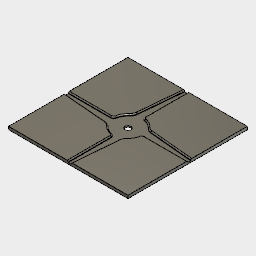
Box Top v3 (Autodesk Fusion 360 design; units mm, degrees)
Autodesk Fusion 360 part; units mm, degrees
sketch "Sketch1" plane through (0, 0, 0) normal (0, 1, 0) x (1, 0, 0)
  line L0 (60, -60) -> (-60, -60)
  line L1 (-60, -60) -> (-60, 60)
  line L2 (-60, 60) -> (60, 60)
  line L3 (60, 60) -> (60, -60)
  line L4 (60, -60) -> (-60, 60) construction
  line L5 (-60, -60) -> (60, 60) construction
  constraint perpendicular L0 L1
  constraint parallel L0 L2
  constraint parallel L1 L3
  constraint horizontal L0
  constraint coincident L4
  constraint coincident L5
extrude "Extrude1" add sketch "Sketch1" along normal blind 3
sketch "Sketch2" plane through (0, 3, 0) normal (0, 1, 0) x (-1, 0, 0)
  line L0 (-60, -60) -> (60, -60)
  line L1 (60, -60) -> (60, 60)
  line L2 (60, 60) -> (-60, 60)
  line L3 (-60, 60) -> (-60, -60)
  circle A0 centre (0, 0) radius 3
  line L4 (0, -60) -> (0, -17.2409)
  line L5 (60, 0) -> (17.4152, 0)
  line L6 (0, 60) -> (0, 16.9303)
  line L7 (-60, 0) -> (-16.7383, 0)
  line L8 (-60, -60) -> (60, -60)
  line L9 (3, -60) -> (7.0006, -16.2997)
  line L10 (60, -60) -> (60, 60)
  line L11 (60, 60) -> (-60, 60)
  line L12 (-60, 60) -> (-60, -60)
  line L13 (-60, -3) -> (-16.05, -7.0235)
  line L14 (60, 3) -> (15.8991, 6.7805)
  line L15 (-2.8992, 60) -> (-6.6949, 15.7222)
  arc A1 (-9.3339, 10.4412) -> (-13.7854, 2.4707) centre (0, 0) ccw
  arc A2 (10.6052, 9.4341) -> (2.4766, 13.9763) centre (0, 0) ccw
  arc A3 (-10.8133, -9.6603) -> (-2.4857, -14.2853) centre (0, 0) ccw
  arc A4 (9.6859, -11.0201) -> (14.4588, -2.4907) centre (0, 0) ccw
  arc A5 (10.6052, 9.4341) -> (15.8991, 6.7805) centre (16.5824, 14.7513) ccw
  arc A6 (9.6859, -11.0201) -> (7.0006, -16.2997) centre (14.9673, -17.029) ccw
  arc A7 (-10.8133, -9.6603) -> (-16.05, -7.0235) centre (-16.7793, -14.9902) ccw
  arc A8 (-9.3339, 10.4412) -> (-6.6949, 15.7222) centre (-14.6657, 16.4055) ccw
  arc A9 (0, -17.2409) -> (-2.4857, -14.2853) centre (-3, -17.2409) ccw
  arc A10 (-16.7383, 0) -> (-13.7854, 2.4707) centre (-16.7383, 3) ccw
  arc A11 (0, 16.9303) -> (2.4766, 13.9763) centre (3, 16.9303) ccw
  arc A12 (17.4152, 0) -> (14.4588, -2.4907) centre (17.4152, -3) ccw
  dimension "d3" = 6
  dimension "d4" = 29
  dimension "d5" = 3
  dimension "d8" = 3
  dimension "d12" = 3
  dimension "d15" = 8
  dimension "d16" = 3
  constraint concentric A0 A3
  constraint midpoint L0
  constraint perpendicular L0 L4
  constraint midpoint L1
  constraint perpendicular L1 L5
  constraint midpoint L2
  constraint perpendicular L2 L6
  constraint midpoint L3
  constraint perpendicular L3 L7
  constraint coincident L0
  constraint coincident L3
  constraint coincident L10
  constraint coincident L11
  constraint perpendicular L14 L15
  constraint concentric A1 A3
  constraint concentric A2 A3
  constraint concentric A3 A4
  constraint tangent L14 A5
  constraint tangent A2 A5
  constraint tangent L9 A6
  constraint tangent A4 A6
  constraint equal A5 A6
  constraint tangent L13 A7
  constraint tangent A3 A7
  constraint equal A5 A7
  constraint tangent L15 A8
  constraint tangent A1 A8
  constraint equal A5 A8
  constraint tangent L4 A9
  constraint tangent A3 A9
  constraint tangent L7 A10
  constraint tangent A1 A10
  constraint equal A9 A10
  constraint tangent L6 A11
  constraint tangent A2 A11
  constraint equal A9 A11
  constraint tangent L5 A12
  constraint tangent A4 A12
  constraint equal A9 A12
  measures "d3" diameter of A0
  measures "d4" diameter of A3
  measures "d15" radius of A5
  measures "d16" radius of A9
extrude "Extrude2" cut sketch "Sketch2" against normal blind 1.5 contours L0 L1 L2 L3 L4 L5 L6 L7 L8 L9 L10 L11 L12 L13 L14 L15 A1 A2 A3 A4 A5 A6 A7 A8 A9 A10 A11 A12
extrude "Extrude3" cut 1 faces at (0.9888, 3, 0.149) along direction (0, -1, 0) blind 10
fillet "Fillet1" radius 1 20 edges at (-38.7076, 3, 0) (-15.4823, 3, -0.7057) (-12.8035, 3, -7.1645) (-7.8366, 3, -13.4022) (-5.0003, 3, -38.1498) (0, 3, 38.4652) (-0.7011, 3, 15.0029) (-6.9239, 3, 12.3907) (-12.9976, 3, 7.5994) (-37.9496, 3, 4.8902) (38.3692, 3, 0) (14.8132, 3, 0.6992) (12.2273, 3, 6.8289) (7.5094, 3, 12.8294) (4.7971, 3, 37.8611) (0, 3, -38.6205) (0.704, 3, -15.31) (7.0402, 3, -12.6762) (13.1814, 3, -7.8449) (38.025, 3, -5.0117)
